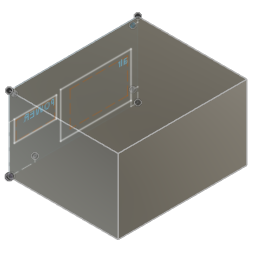
variable PSU (Autodesk Fusion 360 archive; units mm, degrees)
design "PSU"
Autodesk Fusion 360 part; units mm, degrees
sketch "Sketch1" plane through (0, 0, 0) normal (0, 0, 1) x (1, 0, 0)
  line L0 (0, 0) -> (127, 0)
  line L1 (127, 0) -> (127, 150)
  line L2 (127, 150) -> (0, 150)
  line L3 (0, 150) -> (0, 0)
  dimension "d1" = 127
  dimension "d2" = 150
  constraint horizontal L0
  constraint vertical L1
  constraint horizontal L2
  constraint vertical L3
  constraint coincident L0.start L3.end
  measures "d1" distance of L0.start L0.end
  measures "d2" distance of L0.start L2.end
extrude "Extrude1" add sketch "Sketch1" along normal blind 87
sketch "Sketch5" plane through (0, 0, 0) normal (-1, 0, 0) x (0, -1, 0)
  line L0 (-150, 0) -> (0, 0)
  line L1 (0, 0) -> (0, 87)
  line L2 (0, 87) -> (-150, 87)
  line L3 (-150, 87) -> (-150, 0)
  line L4 (-150, 0) -> (-142, 0) construction
  line L5 (-142, 0) -> (-142, 6) construction
  line L6 (-142, 6) -> (-60, 6)
  line L7 (-60, 6) -> (-60, 58)
  line L8 (-60, 58) -> (-142, 58)
  line L9 (-142, 58) -> (-142, 6)
  line L10 (0, 0) -> (0, 55) construction
  line L11 (0, 55) -> (-6, 55) construction
  line L12 (-6, 55) -> (-55, 55)
  line L13 (-55, 55) -> (-55, 31)
  line L14 (-55, 31) -> (-6, 31)
  line L15 (-6, 31) -> (-6, 55)
  line L16 (-53, 32) -> (-8, 32) construction
  line L17 (-8, 32) -> (-8, 53) construction
  line L18 (-8, 53) -> (-53, 53) construction
  line L19 (-53, 53) -> (-53, 32) construction
  line L20 (-138, 13) -> (-71, 13) construction
  line L21 (-71, 13) -> (-71, 53) construction
  line L22 (-71, 53) -> (-138, 53) construction
  line L23 (-138, 53) -> (-138, 13) construction
  line L24 (-150, 0) -> (-150, 16) construction
  line L25 (-150, 16) -> (-144, 16) construction
  circle A0 centre (-144, 16) radius 1.75
  line L26 (-150, 87) -> (-150, 81) construction
  line L27 (-150, 81) -> (-144, 81) construction
  circle A1 centre (-144, 81) radius 1.75
  line L28 (0, 0) -> (-2.473, 0)
  line L29 (0, 0) -> (-30, 0) construction
  line L30 (-30, 0) -> (-30, 6) construction
  circle A2 centre (-30, 6) radius 1.75
  line L31 (0, 87) -> (-6, 87) construction
  line L32 (-6, 87) -> (-6, 81) construction
  circle A3 centre (-6, 81) radius 1.75
  dimension "d18" = 8
  dimension "d19" = 6
  dimension "d20" = 82
  dimension "d21" = 52
  dimension "d26" = 55
  dimension "d27" = 6
  dimension "d28" = 49
  dimension "d29" = 24
  dimension "d30" = 7
  dimension "d31" = 7
  dimension "d51" = 16
  dimension "d52" = 6
  dimension "d53" = 3.5
  dimension "d54" = 6
  dimension "d55" = 3.5
  dimension "d56" = 30
  dimension "d57" = 6
  dimension "d58" = 3.5
  dimension "d59" = 6
  dimension "d60" = 6
  dimension "d61" = 3.5
  constraint coincident L0.start L3.end
  constraint perpendicular L3 L4
  constraint perpendicular L4 L5
  constraint horizontal L6
  constraint vertical L7
  constraint horizontal L8
  constraint vertical L9
  constraint coincident L0.end L1.start
  constraint perpendicular L0 L10
  constraint perpendicular L10 L11
  constraint horizontal L12
  constraint vertical L13
  constraint horizontal L14
  constraint vertical L15
  constraint perpendicular L4 L24
  constraint perpendicular L24 L25
  constraint coincident L25.end A0.centre
  constraint coincident L2.end L3.start
  constraint perpendicular L2 L26
  constraint perpendicular L26 L27
  constraint coincident L27.end A1.centre
  constraint coincident L0 L28.end
  constraint perpendicular L10 L29
  constraint perpendicular L29 L30
  constraint coincident L30.end A2.centre
  constraint coincident L1.end L2.start
  constraint perpendicular L1 L31
  constraint perpendicular L31 L32
  constraint coincident L32.end A3.centre
  measures "d18" distance of L0.start L4.end
  measures "d19" distance of L4.end L5.end
  measures "d20" distance of L5.end L6.end
  measures "d21" distance of L5.end L8.end
  measures "d26" distance of L0.end L10.end
  measures "d27" distance of L10.end L11.end
  measures "d28" distance of L11.end L12.end
  measures "d29" distance of L11.end L14.end
  measures "d51" distance of L0.start L24.end
  measures "d52" distance of L24.end L25.end
  measures "d53" diameter of A0
  measures "d54" distance of L2.end L26.end
  measures "d55" diameter of A1
  measures "d56" distance of L0.end L29.end
  measures "d57" distance of L29.end L30.end
  measures "d58" diameter of A2
  measures "d59" distance of L1.end L31.end
  measures "d60" distance of L31.end L32.end
  measures "d61" diameter of A3
extrude "Extrude3" [suppressed]
extrude "Extrude4" [suppressed]
sketch "Sketch6" plane through (0, 0, 87) normal (0, 0, 1) x (-1, 0, 0)
  line L0 (0, -150) -> (0, 0)
  line L1 (0, 0) -> (-127, 0)
  line L2 (-127, 0) -> (-127, -150)
  line L3 (-127, -150) -> (0, -150)
  line L4 (0, -150) -> (0, -138)
  line L5 (0, -138) -> (-4, -138)
  line L6 (-4, -138) -> (-124, -138)
  line L7 (-124, -138) -> (-124, -18)
  line L8 (-124, -18) -> (-4, -18)
  line L9 (-4, -18) -> (-4, -138)
  line L10 (-26.1497, -102.2792) -> (-26.1497, -39.2792) construction
  line L11 (-26.1497, -39.2792) -> (-78.1497, -39.2792) construction
  line L12 (-78.1497, -39.2792) -> (-78.1497, -102.2792) construction
  line L13 (-78.1497, -102.2792) -> (-26.1497, -102.2792) construction
  dimension "d36" = 12
  dimension "d37" = 4
  dimension "d38" = 120
  dimension "d39" = 120
  dimension "d42" = 12
  constraint coincident L0.start L3.end
  constraint perpendicular L3 L4
  constraint perpendicular L4 L5
  constraint horizontal L6
  constraint vertical L7
  constraint horizontal L8
  constraint vertical L9
  measures "d36" distance of L0.start L4.end
  measures "d37" distance of L4.end L5.end
  measures "d38" distance of L5.end L6.end
  measures "d39" distance of L5.end L8.end
extrude "Extrude5" [suppressed]
extrude "Extrude6" [suppressed]
sketch "Sketch7" plane through (127, 0, 0) normal (1, 0, 0) x (0, 1, 0)
  line L0 (0, 0) -> (150, 0)
  line L1 (150, 0) -> (150, 87)
  line L2 (150, 87) -> (0, 87)
  line L3 (0, 87) -> (0, 0)
  circle A0 centre (20, 40) radius 17
  line L4 (9, 33) -> (29, 33) construction
  line L5 (29, 33) -> (29, 46) construction
  line L6 (29, 46) -> (9, 46) construction
  line L7 (9, 46) -> (9, 33) construction
  dimension "d45" = 34
  dimension "d48" = 7
  measures "d45" diameter of A0
extrude "Extrude7" [suppressed]
extrude "Extrude8" [suppressed]
extrude "Extrude9" [suppressed]
equation "d51 = 15 mm + 1 mm"
equation "d52 = 5 mm + 1 mm"
